Autodesk Inventor part; units mm, degrees
(part 2 of 2)
sketch "DXF" plane through (0, 0, 0) normal (0, 0, 1) x (1, 0, 0)
  arc A0 (1.0814, 45.4571) -> (-1.0814, 45.4571) centre (0, 0) ccw
  arc A1 (2.6745, 40.3222) -> (1.0814, 45.4571) centre (-21.6776, 35.5812) ccw
  arc A2 (3.9987, 40.2125) -> (2.6745, 40.3222) centre (0, 0) ccw
  arc A3 (6.4154, 45.0151) -> (3.9987, 40.2125) centre (27.2384, 31.5279) ccw
  arc A4 (8.5486, 44.6592) -> (6.4154, 45.0151) centre (0, 0) ccw
  arc A5 (9.2749, 39.3321) -> (8.5486, 44.6592) centre (-15.5255, 38.6639) ccw
  arc A6 (10.563, 39.0059) -> (9.2749, 39.3321) centre (0, 0) ccw
  arc A7 (13.7371, 43.3453) -> (10.563, 39.0059) centre (32.0562, 26.6146) ccw
  arc A8 (15.7827, 42.643) -> (13.7371, 43.3453) centre (0, 0) ccw
  arc A9 (15.6222, 37.269) -> (15.7827, 42.643) centre (-8.9499, 40.692) ccw
  arc A10 (16.8391, 36.7353) -> (15.6222, 37.269) centre (0, 0) ccw
  arc A11 (20.6842, 40.493) -> (16.8391, 36.7353) centre (35.9996, 20.9753) ccw
  arc A12 (22.5862, 39.4637) -> (20.6842, 40.493) centre (0, 0) ccw
  arc A13 (21.5435, 34.1894) -> (22.5862, 39.4637) centre (-2.1301, 41.6101) ccw
  arc A14 (22.6558, 33.4627) -> (21.5435, 34.1894) centre (0, 0) ccw
  arc A15 (27.067, 36.5363) -> (22.6558, 33.4627) centre (38.9611, 14.7639) ccw
  arc A16 (28.7737, 35.2079) -> (27.067, 36.5363) centre (0, 0) ccw
  arc A17 (26.877, 30.1772) -> (28.7737, 35.2079) centre (4.7477, 41.3932) ccw
  arc A18 (27.8546, 29.2772) -> (26.877, 30.1772) centre (0, 0) ccw
  arc A19 (32.7115, 31.5829) -> (27.8546, 29.2772) centre (40.8598, 8.1497) ccw
  arc A20 (34.1763, 29.9917) -> (32.7115, 31.5829) centre (0, 0) ccw
  arc A21 (31.4775, 25.3418) -> (34.1763, 29.9917) centre (11.4961, 40.0472) ccw
  arc A22 (32.2936, 24.2932) -> (31.4775, 25.3418) centre (0, 0) ccw
  arc A23 (37.4637, 25.768) -> (32.2936, 24.2932) centre (41.6439, 1.3133) ccw
  arc A24 (38.6466, 23.9574) -> (37.4637, 25.768) centre (0, 0) ccw
  arc A25 (35.2193, 19.8151) -> (38.6466, 23.9574) centre (17.9308, 37.6088) ccw
  arc A26 (35.8517, 18.6465) -> (35.2193, 19.8151) centre (0, 0) ccw
  arc A27 (41.1941, 19.2502) -> (35.8517, 18.6465) centre (41.2921, -5.559) ccw
  arc A28 (42.0628, 17.2696) -> (41.1941, 19.2502) centre (0, 0) ccw
  arc A29 (38.0004, 13.748) -> (42.0628, 17.2696) centre (23.8765, 34.1446) ccw
  arc A30 (38.4318, 12.4912) -> (38.0004, 13.748) centre (0, 0) ccw
  arc A31 (43.8007, 12.2073) -> (38.4318, 12.4912) centre (39.8139, -12.2796) ccw
  arc A32 (44.3316, 10.1108) -> (43.8007, 12.2073) centre (0, 0) ccw
  arc A33 (39.745, 7.3058) -> (44.3316, 10.1108) centre (29.1709, 29.7489) ccw
  arc A34 (39.9637, 5.9952) -> (39.745, 7.3058) centre (0, 0) ccw
  arc A35 (45.2126, 4.8315) -> (39.9637, 5.9952) centre (37.2498, -18.6653) ccw
  arc A36 (45.3912, 2.6762) -> (45.2126, 4.8315) centre (0, 0) ccw
  arc A37 (40.4054, 0.6644) -> (45.3912, 2.6762) centre (33.6695, 24.5418) ccw
  arc A38 (40.4054, -0.6644) -> (40.4054, 0.6644) centre (0, 0) ccw
  arc A39 (45.3912, -2.6762) -> (40.4054, -0.6644) centre (33.6695, -24.5418) ccw
  arc A40 (45.2126, -4.8315) -> (45.3912, -2.6762) centre (0, 0) ccw
  arc A41 (39.9637, -5.9952) -> (45.2126, -4.8315) centre (37.2498, 18.6653) ccw
  arc A42 (39.745, -7.3058) -> (39.9637, -5.9952) centre (0, 0) ccw
  arc A43 (44.3316, -10.1108) -> (39.745, -7.3058) centre (29.1709, -29.7489) ccw
  arc A44 (43.8007, -12.2073) -> (44.3316, -10.1108) centre (0, 0) ccw
  arc A45 (38.4318, -12.4912) -> (43.8007, -12.2073) centre (39.8139, 12.2796) ccw
  arc A46 (38.0004, -13.748) -> (38.4318, -12.4912) centre (0, 0) ccw
  arc A47 (42.0628, -17.2696) -> (38.0004, -13.748) centre (23.8765, -34.1446) ccw
  arc A48 (41.1941, -19.2502) -> (42.0628, -17.2696) centre (0, 0) ccw
  arc A49 (35.8517, -18.6465) -> (41.1941, -19.2502) centre (41.2921, 5.559) ccw
  arc A50 (35.2193, -19.8151) -> (35.8517, -18.6465) centre (0, 0) ccw
  arc A51 (38.6466, -23.9574) -> (35.2193, -19.8151) centre (17.9308, -37.6088) ccw
  arc A52 (37.4637, -25.768) -> (38.6466, -23.9574) centre (0, 0) ccw
  arc A53 (32.2936, -24.2932) -> (37.4637, -25.768) centre (41.6439, -1.3133) ccw
  arc A54 (31.4775, -25.3418) -> (32.2936, -24.2932) centre (0, 0) ccw
  arc A55 (34.1763, -29.9917) -> (31.4775, -25.3418) centre (11.4961, -40.0472) ccw
  arc A56 (32.7115, -31.5829) -> (34.1763, -29.9917) centre (0, 0) ccw
  arc A57 (27.8546, -29.2772) -> (32.7115, -31.5829) centre (40.8598, -8.1497) ccw
  arc A58 (26.877, -30.1772) -> (27.8546, -29.2772) centre (0, 0) ccw
  arc A59 (28.7737, -35.2079) -> (26.877, -30.1772) centre (4.7477, -41.3932) ccw
  arc A60 (27.067, -36.5363) -> (28.7737, -35.2079) centre (0, 0) ccw
  arc A61 (22.6558, -33.4627) -> (27.067, -36.5363) centre (38.9611, -14.7639) ccw
  arc A62 (21.5435, -34.1894) -> (22.6558, -33.4627) centre (0, 0) ccw
  arc A63 (22.5862, -39.4637) -> (21.5435, -34.1894) centre (-2.1301, -41.6101) ccw
  arc A64 (20.6842, -40.493) -> (22.5862, -39.4637) centre (0, 0) ccw
  arc A65 (16.8391, -36.7353) -> (20.6842, -40.493) centre (35.9996, -20.9753) ccw
  arc A66 (15.6222, -37.269) -> (16.8391, -36.7353) centre (0, 0) ccw
  arc A67 (15.7827, -42.643) -> (15.6222, -37.269) centre (-8.9499, -40.692) ccw
  arc A68 (13.7371, -43.3453) -> (15.7827, -42.643) centre (0, 0) ccw
  arc A69 (10.563, -39.0059) -> (13.7371, -43.3453) centre (32.0562, -26.6146) ccw
  arc A70 (9.2749, -39.3321) -> (10.563, -39.0059) centre (0, 0) ccw
  arc A71 (8.5486, -44.6592) -> (9.2749, -39.3321) centre (-15.5255, -38.6639) ccw
  arc A72 (6.4154, -45.0151) -> (8.5486, -44.6592) centre (0, 0) ccw
  arc A73 (3.9987, -40.2125) -> (6.4154, -45.0151) centre (27.2384, -31.5279) ccw
  arc A74 (2.6745, -40.3222) -> (3.9987, -40.2125) centre (0, 0) ccw
  arc A75 (1.0814, -45.4571) -> (2.6745, -40.3222) centre (-21.6776, -35.5812) ccw
  arc A76 (-1.0814, -45.4571) -> (1.0814, -45.4571) centre (0, 0) ccw
  arc A77 (-2.6745, -40.3222) -> (-1.0814, -45.4571) centre (21.6776, -35.5812) ccw
  arc A78 (-3.9987, -40.2125) -> (-2.6745, -40.3222) centre (0, 0) ccw
  arc A79 (-6.4154, -45.0151) -> (-3.9987, -40.2125) centre (-27.2384, -31.5279) ccw
  arc A80 (-8.5486, -44.6592) -> (-6.4154, -45.0151) centre (0, 0) ccw
  arc A81 (-9.2749, -39.3321) -> (-8.5486, -44.6592) centre (15.5255, -38.6639) ccw
  arc A82 (-10.563, -39.0059) -> (-9.2749, -39.3321) centre (0, 0) ccw
  arc A83 (-13.7371, -43.3453) -> (-10.563, -39.0059) centre (-32.0562, -26.6146) ccw
  arc A84 (-15.7827, -42.643) -> (-13.7371, -43.3453) centre (0, 0) ccw
  arc A85 (-15.6222, -37.269) -> (-15.7827, -42.643) centre (8.9499, -40.692) ccw
  arc A86 (-16.8391, -36.7353) -> (-15.6222, -37.269) centre (0, 0) ccw
  arc A87 (-20.6842, -40.493) -> (-16.8391, -36.7353) centre (-35.9996, -20.9753) ccw
  arc A88 (-22.5862, -39.4637) -> (-20.6842, -40.493) centre (0, 0) ccw
  arc A89 (-21.5435, -34.1894) -> (-22.5862, -39.4637) centre (2.1301, -41.6101) ccw
  arc A90 (-22.6558, -33.4627) -> (-21.5435, -34.1894) centre (0, 0) ccw
  arc A91 (-27.067, -36.5363) -> (-22.6558, -33.4627) centre (-38.9611, -14.7639) ccw
  arc A92 (-28.7737, -35.2079) -> (-27.067, -36.5363) centre (0, 0) ccw
  arc A93 (-26.877, -30.1772) -> (-28.7737, -35.2079) centre (-4.7477, -41.3932) ccw
  arc A94 (-27.8546, -29.2772) -> (-26.877, -30.1772) centre (0, 0) ccw
  arc A95 (-32.7115, -31.5829) -> (-27.8546, -29.2772) centre (-40.8598, -8.1497) ccw
  arc A96 (-34.1763, -29.9917) -> (-32.7115, -31.5829) centre (0, 0) ccw
  arc A97 (-31.4775, -25.3418) -> (-34.1763, -29.9917) centre (-11.4961, -40.0472) ccw
  arc A98 (-32.2936, -24.2932) -> (-31.4775, -25.3418) centre (0, 0) ccw
  arc A99 (-37.4637, -25.768) -> (-32.2936, -24.2932) centre (-41.6439, -1.3133) ccw
  arc A100 (-38.6466, -23.9574) -> (-37.4637, -25.768) centre (0, 0) ccw
  arc A101 (-35.2193, -19.8151) -> (-38.6466, -23.9574) centre (-17.9308, -37.6088) ccw
  arc A102 (-35.8517, -18.6465) -> (-35.2193, -19.8151) centre (0, 0) ccw
  arc A103 (-41.1941, -19.2502) -> (-35.8517, -18.6465) centre (-41.2921, 5.559) ccw
  arc A104 (-42.0628, -17.2696) -> (-41.1941, -19.2502) centre (0, 0) ccw
  arc A105 (-38.0004, -13.748) -> (-42.0628, -17.2696) centre (-23.8765, -34.1446) ccw
  arc A106 (-38.4318, -12.4912) -> (-38.0004, -13.748) centre (0, 0) ccw
  arc A107 (-43.8007, -12.2073) -> (-38.4318, -12.4912) centre (-39.8139, 12.2796) ccw
  arc A108 (-44.3316, -10.1108) -> (-43.8007, -12.2073) centre (0, 0) ccw
  arc A109 (-39.745, -7.3058) -> (-44.3316, -10.1108) centre (-29.1709, -29.7489) ccw
  arc A110 (-39.9637, -5.9952) -> (-39.745, -7.3058) centre (0, 0) ccw
  arc A111 (-45.2126, -4.8315) -> (-39.9637, -5.9952) centre (-37.2498, 18.6653) ccw
  arc A112 (-45.3912, -2.6762) -> (-45.2126, -4.8315) centre (0, 0) ccw
  arc A113 (-40.4054, -0.6644) -> (-45.3912, -2.6762) centre (-33.6695, -24.5418) ccw
  arc A114 (-40.4054, 0.6644) -> (-40.4054, -0.6644) centre (0, 0) ccw
  arc A115 (-45.3912, 2.6762) -> (-40.4054, 0.6644) centre (-33.6695, 24.5418) ccw
  arc A116 (-45.2126, 4.8315) -> (-45.3912, 2.6762) centre (0, 0) ccw
  arc A117 (-39.9637, 5.9952) -> (-45.2126, 4.8315) centre (-37.2498, -18.6653) ccw
  arc A118 (-39.745, 7.3058) -> (-39.9637, 5.9952) centre (0, 0) ccw
  arc A119 (-44.3316, 10.1108) -> (-39.745, 7.3058) centre (-29.1709, 29.7489) ccw
  arc A120 (-43.8007, 12.2073) -> (-44.3316, 10.1108) centre (0, 0) ccw
  arc A121 (-38.4318, 12.4912) -> (-43.8007, 12.2073) centre (-39.8139, -12.2796) ccw
  arc A122 (-38.0004, 13.748) -> (-38.4318, 12.4912) centre (0, 0) ccw
  arc A123 (-42.0628, 17.2696) -> (-38.0004, 13.748) centre (-23.8765, 34.1446) ccw
  arc A124 (-41.1941, 19.2502) -> (-42.0628, 17.2696) centre (0, 0) ccw
  arc A125 (-35.8517, 18.6465) -> (-41.1941, 19.2502) centre (-41.2921, -5.559) ccw
  arc A126 (-35.2193, 19.8151) -> (-35.8517, 18.6465) centre (0, 0) ccw
  arc A127 (-38.6466, 23.9574) -> (-35.2193, 19.8151) centre (-17.9308, 37.6088) ccw
  arc A128 (-37.4637, 25.768) -> (-38.6466, 23.9574) centre (0, 0) ccw
  arc A129 (-32.2936, 24.2932) -> (-37.4637, 25.768) centre (-41.6439, 1.3133) ccw
  arc A130 (-31.4775, 25.3418) -> (-32.2936, 24.2932) centre (0, 0) ccw
  arc A131 (-34.1763, 29.9917) -> (-31.4775, 25.3418) centre (-11.4961, 40.0472) ccw
  arc A132 (-32.7115, 31.5829) -> (-34.1763, 29.9917) centre (0, 0) ccw
  arc A133 (-27.8546, 29.2772) -> (-32.7115, 31.5829) centre (-40.8598, 8.1497) ccw
  arc A134 (-26.877, 30.1772) -> (-27.8546, 29.2772) centre (0, 0) ccw
  arc A135 (-28.7737, 35.2079) -> (-26.877, 30.1772) centre (-4.7477, 41.3932) ccw
  arc A136 (-27.067, 36.5363) -> (-28.7737, 35.2079) centre (0, 0) ccw
  arc A137 (-22.6558, 33.4627) -> (-27.067, 36.5363) centre (-38.9611, 14.7639) ccw
  arc A138 (-21.5435, 34.1894) -> (-22.6558, 33.4627) centre (0, 0) ccw
  arc A139 (-22.5862, 39.4637) -> (-21.5435, 34.1894) centre (2.1301, 41.6101) ccw
  arc A140 (-20.6842, 40.493) -> (-22.5862, 39.4637) centre (0, 0) ccw
  arc A141 (-16.8391, 36.7353) -> (-20.6842, 40.493) centre (-35.9996, 20.9753) ccw
  arc A142 (-15.6222, 37.269) -> (-16.8391, 36.7353) centre (0, 0) ccw
  arc A143 (-15.7827, 42.643) -> (-15.6222, 37.269) centre (8.9499, 40.692) ccw
  arc A144 (-13.7371, 43.3453) -> (-15.7827, 42.643) centre (0, 0) ccw
  arc A145 (-10.563, 39.0059) -> (-13.7371, 43.3453) centre (-32.0562, 26.6146) ccw
  arc A146 (-9.2749, 39.3321) -> (-10.563, 39.0059) centre (0, 0) ccw
  arc A147 (-8.5486, 44.6592) -> (-9.2749, 39.3321) centre (15.5255, 38.6639) ccw
  arc A148 (-6.4154, 45.0151) -> (-8.5486, 44.6592) centre (0, 0) ccw
  arc A149 (-3.9987, 40.2125) -> (-6.4154, 45.0151) centre (-27.2384, 31.5279) ccw
  arc A150 (-2.6745, 40.3222) -> (-3.9987, 40.2125) centre (0, 0) ccw
  arc A151 (-1.0814, 45.4571) -> (-2.6745, 40.3222) centre (21.6776, 35.5812) ccw
  circle A152 centre (-12, 12) radius 2.72
  circle A153 centre (0, 0) radius 5.22
  circle A154 centre (-12, -12) radius 2.72
  circle A155 centre (12, 12) radius 2.72
  circle A156 centre (12, -12) radius 2.72
equation "\"d0\" = da_da"
equation "\"d1\" = da_b"
equation "\"d3\" = da_dw"
equation "\"da_da\" = 90.5"
equation "\"da_b\" = 20"
equation "\"da_dw\" = 85.806452"
body "Solid1"
body "Srf1"
